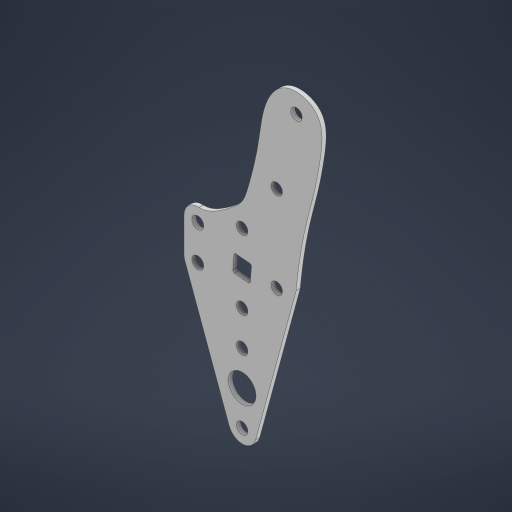
# Autodesk Inventor part: coffin-v2
Saved by Autodesk Inventor 2023.2 (Build 272271000, 271)
## iProperties
Created: 2023-04-01
Part Number: coffin-v2
Material: Generic
Document SubType Name: Modeling
Designer: Liam
Density: 1 g/cm^3
Appearance: Default
Author: Liam
Autodesk Inventor part; units mm, degrees
ref_plane "YZ Plane" through (0, 0, 0) normal (1, 0, 0) x (0, 1, 0)
ref_plane "XZ Plane" through (0, 0, 0) normal (0, 1, 0) x (-1, 0, 0)
ref_plane "XY Plane" through (0, 0, 0) normal (0, 0, 1) x (1, 0, 0)
sketch "Sketch1" plane through (0, 0, 0) normal (0, 0, 1) x (1, 0, 0)
  line L0 (37.223, 2.7469) -> (22.3469, -52.1291)
  arc A0 (12.6742, -52.5484) -> (22.3469, -52.1291) centre (17.4439, -50.8) ccw
  line L1 (12.6742, -52.5484) -> (-3.6199, -8.0984)
  arc A1 (-3.9302, -6.35) -> (-3.6199, -8.0984) centre (1.1498, -6.35) ccw
  line L2 (-3.9302, -6.35) -> (-3.9302, 6.35)
  arc A2 (1.5775, 11.412) -> (-3.9302, 6.35) centre (1.1498, 6.35) ccw
  arc A3 (20.8415, 2.2589) -> (20.2651, 2.9475) centre (20.209, 2.315) ccw
  line L3 (20.2651, 2.9475) -> (15.185, 3.3976)
  arc A4 (15.185, 3.3976) -> (14.4964, 2.8212) centre (15.1289, 2.7651) ccw
  line L4 (14.4964, 2.8212) -> (14.0462, -2.2589)
  arc A5 (14.0462, -2.2589) -> (14.6227, -2.9475) centre (14.6788, -2.315) ccw
  line L5 (14.6227, -2.9475) -> (19.7028, -3.3976)
  arc A6 (19.7028, -3.3976) -> (20.3914, -2.8212) centre (19.7589, -2.7651) ccw
  line L6 (20.3914, -2.8212) -> (20.8415, 2.2589)
  circle A7 centre (17.4439, -38.1) radius 5.08
  circle A8 centre (17.4439, -25.4) radius 2.1082
  circle A9 centre (17.4439, -12.7) radius 2.1082
  circle A10 centre (30.1439, 0) radius 2.1082
  circle A11 centre (17.4439, 12.7) radius 2.1082
  circle A12 centre (1.1498, 6.35) radius 2.1844
  circle A13 centre (1.1498, -6.35) radius 2.1844
  circle A14 centre (17.4439, -50.8) radius 2.0955
  circle A15 centre (37.3901, 58.9556) radius 2.0955
  line L7 (1.5775, 11.412) -> (5.589, 11.073) construction
  line L8 (5.589, 11.073) -> (15.3484, 18.7863) construction
  line L9 (15.3484, 18.7863) -> (18.0418, 20.7541) construction
  line L10 (18.0418, 20.7541) -> (19.8489, 27.8291) construction
  line L11 (19.8489, 27.8291) -> (23.8326, 41.9032) construction
  line L12 (23.8326, 41.9032) -> (24.3915, 54.927) construction
  line L13 (24.3915, 54.927) -> (29.8719, 65.007) construction
  line L14 (29.8719, 65.007) -> (37.691, 67.16) construction
  line L15 (37.691, 67.16) -> (46.1173, 63.8326) construction
  line L16 (46.1173, 63.8326) -> (47.3895, 55.8078) construction
  line L17 (47.3895, 55.8078) -> (45.4323, 45.1406) construction
  line L18 (45.4323, 45.1406) -> (43.5728, 34.5713) construction
  line L19 (43.5728, 34.5713) -> (38.6988, 19.4023) construction
  line L20 (38.6988, 19.4023) -> (37.223, 2.7469) construction
  line L21 (37.223, 2.7469) -> (37.223, 2.7469) construction
  spline S0 degree 4 poles (1.5775, 11.412) (5.589, 11.073) (15.3484, 18.7863) (18.0418, 20.7541) (19.8489, 27.8291) (23.8326, 41.9032) (24.3915, 54.927) (29.8719, 65.007) (37.691, 67.16) (46.1173, 63.8326) (47.3895, 55.8078) (45.4323, 45.1406) (43.5728, 34.5713) (38.6988, 19.4023) (37.2245, 2.7635) (37.223, 2.7469) knots 1 1 1 1 1 2 3 4 5 6 7 8 9 10 11 12 13 13 13 13 13
  circle A16 centre (30.1439, 31.5888) radius 2.0955
  point P0 (-3.9302, 6.35)
  point P1 (-3.9302, -6.35)
  point P2 (-3.6199, -8.0984)
  point P3 (12.6742, -52.5484)
  point P4 (21.7462, -53.5011)
  point P5 (20.8415, 2.2589)
  point P6 (20.3914, -2.8212)
  point P7 (14.6227, -2.9475)
  point P8 (14.4964, 2.8212)
  point P9 (20.2651, 2.9475)
  dimension "d0" = 4.3688
  dimension "d1" = 4.3688
  dimension "d2" = 4.2164
  dimension "d3" = 4.2164
  dimension "d5" = 4.2164
  dimension "d6" = 4.2164
  dimension "d7" = 10.16
  dimension "d8" = 4.191
  dimension "d11" = 4.191
  dimension "d12" = 4.191
  constraints: 17 centre point, 14 end point, 14 point on circle, 1 coincident, 1 horizontal, 1 tangent, 28 other
  measures "d0" diameter of A12
  measures "d1" diameter of A13
  measures "d2" diameter of A11
  measures "d3" diameter of A10
  measures "d5" diameter of A9
  measures "d6" diameter of A8
  measures "d7" diameter of A7
  measures "d8" diameter of A14
  measures "d11" diameter of A15
  measures "d12" diameter of A16
extrude "Extrusion1" add sketch "Sketch1" along normal blind 1.524
body "Solid1"
